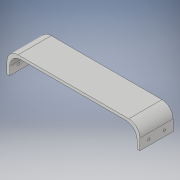
# Autodesk Inventor part: Bumper
Saved by Autodesk Inventor 2019 (Build 230136000, 136)
## iProperties
Created: 2018-12-25
Part Number: Bumper
Material: Generic
Document SubType Name: Modeling
Designer: Martin
Density: 1 g/cm^3
Appearance: Default
Mass: 13.0936 g
Surface Area: 105.326 cm^2
Volume: 13.0936 cm^3
Author: Martin
Autodesk Inventor part; units mm, degrees
ref_plane "YZ Plane" through (0, 0, 0) normal (1, 0, 0) x (0, 1, 0)
ref_plane "XZ Plane" through (0, 0, 0) normal (0, 1, 0) x (-1, 0, 0)
ref_plane "XY Plane" through (0, 0, 0) normal (0, 0, 1) x (1, 0, 0)
sketch "Sketch1" plane through (0, 0, 0) normal (0, 0, 1) x (1, 0, 0)
  line L0 (60, 10) -> (-60, 10)
  line L1 (-60, 10) -> (-60, -10)
  line L2 (60, -10) -> (60, 10)
  line L3 (60, 10) -> (-60, -10) construction
  line L4 (-60, 10) -> (60, -10) construction
  line L5 (57.5, 7.5) -> (-57.5, 7.5)
  line L6 (-57.5, 7.5) -> (-57.5, -10)
  line L7 (57.5, -10) -> (57.5, 7.5)
  line L8 (-60, -10) -> (-57.5, -10)
  line L9 (57.5, -10) -> (60, -10)
  point P0 (0, 0)
  dimension "d0" = 120
  dimension "d1" = 20
  dimension "d14" = 2.5
  dimension "d15" = 2.5
  dimension "d16" = 20
  dimension "d17" = 2.5
  constraints: 20 end point, 4 parallel, 2 midpoint, 2 perpendicular, 1 horizontal
  measures "d0" distance of L2.start L1.end
  measures "d1" distance of L1.end L0.end
  measures "d14" distance between parallel lines of L5 L0
  measures "d15" distance between parallel lines of L6 L1
  measures "d16" distance between parallel lines of L9 L0
  measures "d17" distance of L7.start L2.start
extrude "Extrusion1" add sketch "Sketch1" along normal blind 30
fillet "Fillet1" radius 10 4 edges at (60, 10, 15) (-60, 10, 15) (-57.5, 7.5, 15) (57.5, 7.5, 15)
sketch "Sketch2" plane through (-60, -10, 0) normal (-1, 0, 0) x (0, 0, 1)
  line L0 (33.379, 5) -> (-9.3676, 5) construction
  line L1 (0, 0) -> (30, 0) projected
  line L2 (22, 36.2118) -> (22, -4.5967) construction
  line L3 (8, 36.2118) -> (8, -2.8739) construction
  line L4 (30, 10) -> (30, 0) construction
  line L5 (0, 10) -> (0, 0) construction
  circle A0 centre (22, 5) radius 1
  circle A1 centre (8, 5) radius 1
  point P0 (0, 10)
  dimension "d7" = 5
  dimension "d8" = 8
  dimension "d9" = 8
  dimension "d10" = 2
  dimension "d11" = 2
  constraints: 6 end point, 4 point on line, 2 centre point, 2 vertical, 1 horizontal
  measures "d7" distance between parallel lines of L1 L0
  measures "d8" distance between parallel lines of L2 L4
  measures "d9" distance between parallel lines of L5 L3
  measures "d10" diameter of A0
  measures "d11" diameter of A1
extrude "Extrusion2" cut sketch "Sketch2" against normal blind 120
equation "\"d16\" = d1"
equation "\"d17\" = d15"
equation "\"d8\" = d9"
body "Solid1"
